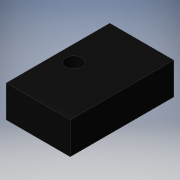
# Autodesk Inventor part: Motor Black Box
Saved by Autodesk Inventor 2016 (Build 200138000, 138)
## iProperties
Created: 2015-06-04
Part Number: Motor Black Box
Material: Stainless Steel
Document SubType Name: Modeling
Designer: Dennis
Density: 8 g/cm^3
Appearance: Glossy - Black
Author: Dennis
Autodesk Inventor part; units mm, degrees
ref_plane "YZ Plane" through (0, 0, 0) normal (1, 0, 0) x (0, 1, 0)
ref_plane "XZ Plane" through (0, 0, 0) normal (0, 1, 0) x (-1, 0, 0)
ref_plane "XY Plane" through (0, 0, 0) normal (0, 0, 1) x (1, 0, 0)
sketch "Sketch1" plane through (0, 0, 0) normal (0, 1, 0) x (-1, 0, 0)
  line L0 (-25.4, 41.0981) -> (25.4, 41.0981)
  line L1 (25.4, 41.0981) -> (25.4, -41.0981)
  line L2 (25.4, -41.0981) -> (-25.4, -41.0981)
  line L3 (-25.4, -41.0981) -> (-25.4, 41.0981)
  line L4 (-25.4, 41.0981) -> (25.4, -41.0981) construction
  line L5 (25.4, 41.0981) -> (-25.4, -41.0981) construction
  circle A0 centre (12.7, 0) radius 6.35
  line L6 (0, 0) -> (12.7, 0) construction
  dimension "d0" = 50.8
  dimension "d1" = 82.1961
  dimension "d2" = 12.7
  dimension "d3" = 12.7
  constraints: 14 end point, 2 horizontal, 2 midpoint, 2 parallel, 1 centre point, 1 perpendicular
  measures "d0" distance of L1.end L2.end
  measures "d1" distance of L0.end L1.end
  measures "d2" distance of L6.start L6.end
  measures "d3" diameter of A0
extrude "Extrusion1" add sketch "Sketch1" along normal blind 25.4
body "Solid1"
